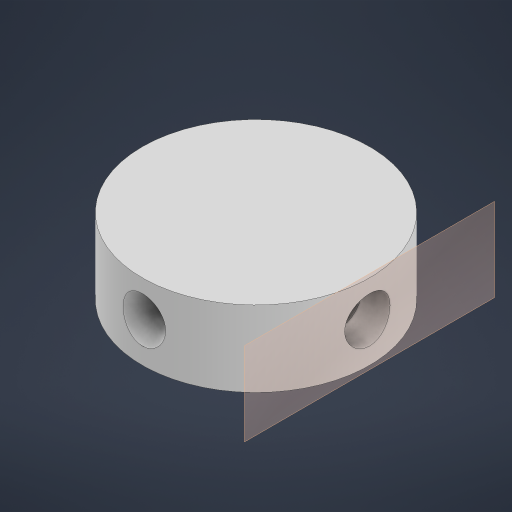
# Autodesk Inventor part: vasen-gewinde-test
Saved by Autodesk Inventor 2023 (Build 270158000, 158)
## iProperties
Created: 2022-06-17
Part Number: vasen-gewinde-test
Material: Generic
Document SubType Name: Modeling
Designer: bananenbrot
Density: 1 g/cm^3
Appearance: Default
Author: bananenbrot
Autodesk Inventor part; units mm, degrees
ref_plane "XZ Plane" through (0, 0, 0) normal (0, 1, 0) x (-1, 0, 0)
ref_plane "XY Plane" through (0, 0, 0) normal (0, 0, 1) x (1, 0, 0)
sketch "Sketch1" plane through (0, 0, 0) normal (0, 1, 0) x (-1, 0, 0)
  circle A0 centre (0, 0) radius 15
  dimension "d0" = 30
  constraints: 1 centre point, 1 coincident
  measures "d0" diameter of A0
extrude "Extrusion1" add sketch "Sketch1" along normal blind 10
ref_plane "Work Plane1" through (15, 0, 0) normal (1, 0, 0) x (0, 1, 0)
sketch "Sketch2" plane through (15, 0, 0) normal (1, 0, 0) x (0, 1, 0)
  circle A0 centre (5.2073, 0) radius 3
  point P0 (0, 0)
  dimension "d4" = 6
  constraints: 1 centre point
  measures "d4" diameter of A0
extrude "Extrusion2" cut sketch "Sketch2" against normal blind 4
pattern_circular "Circular Pattern1" count 4 over 360 about axis through (0, -10, 0) along (0, 1, 0) of "Extrusion2"
chamfer "Chamfer1" distance 3.99 distance2 1 1 edges at (0, 2.2073, -11) measured on face at (0, 2.2073, -11.5)
chamfer "Chamfer2" distance 3.99 distance2 2 1 edges at (-11, 2.2073, 0) measured on face at (-11.5, 2.2073, 0)
chamfer "Chamfer3" distance 3.99 distance2 3 1 edges at (0, 2.2073, 11) measured on face at (0, 2.2073, 11.5)
body "Solid1"
